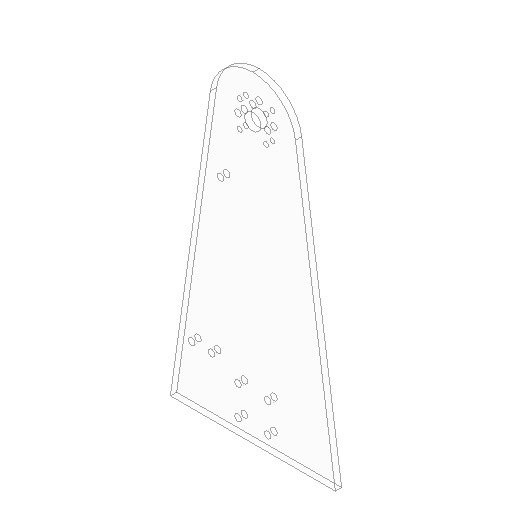
# Autodesk Inventor part: Columna
Saved by Autodesk Inventor 2025.3 (Build 293356000, 356)
## iProperties
Created: 2025-11-11
Part Number: Columna
Material: PMMA Plastic
Document SubType Name: Modeling
Designer: Gabriel Bojaca
Density: 1.188 g/cm^3
Appearance: Polycarbonate - Clear
Author: Gabriel Bojaca
Autodesk Inventor part; units mm, degrees
ref_plane "YZ Plane" through (0, 0, 0) normal (1, 0, 0) x (0, 1, 0)
ref_plane "XZ Plane" through (0, 0, 0) normal (0, 1, 0) x (-1, 0, 0)
ref_plane "XY Plane" through (0, 0, 0) normal (0, 0, 1) x (1, 0, 0)
sketch "Sketch3" plane through (0, 0, 0) normal (0, 0, 1) x (1, 0, 0)
  line L0 (0, 0) -> (100, 0)
  line L1 (100, 0) -> (100, 195) construction
  line L2 (100, 195) -> (0, 195) construction
  line L3 (0, 195) -> (0, 0) construction
  line L4 (50, 0) -> (50, 169) construction
  circle A0 centre (50, 169) radius 4.95
  line L5 (42, 161) -> (58, 161) construction
  line L6 (58, 161) -> (58, 177) construction
  line L7 (58, 177) -> (42, 177) construction
  line L8 (42, 177) -> (42, 161) construction
  line L9 (42, 161) -> (58, 177) construction
  line L10 (58, 161) -> (42, 177) construction
  circle A1 centre (42, 177) radius 1.5
  circle A2 centre (58, 177) radius 1.5
  circle A3 centre (42, 161) radius 1.5
  circle A4 centre (58, 161) radius 1.5
  line L11 (0, 0) -> (24.1871, 172.1)
  line L12 (0, 0) -> (268.3215, 0) construction
  line L13 (100, 0) -> (75.8129, 172.1)
  line L14 (0, 172.1) -> (100, 172.1) construction
  arc A5 (50, 195) -> (24.1871, 172.1) centre (50.5367, 168.3968) ccw
  arc A6 (75.8129, 172.1) -> (50, 195) centre (49.4633, 168.3968) ccw
  line L15 (50, 169) -> (59, 169) construction
  line L16 (50, 169) -> (41, 169) construction
  circle A7 centre (59, 169) radius 2
  circle A8 centre (41, 169) radius 2
  line L17 (41, 9) -> (59, 9) construction
  line L18 (59, 9) -> (59, 27) construction
  line L19 (59, 27) -> (41, 27) construction
  line L20 (41, 27) -> (41, 9) construction
  line L21 (41, 9) -> (59, 27) construction
  line L22 (59, 9) -> (41, 27) construction
  circle A9 centre (41, 27) radius 2
  circle A10 centre (41, 9) radius 2
  circle A11 centre (59, 27) radius 2
  circle A12 centre (59, 9) radius 2
  line L23 (50, 169) -> (50, 178) construction
  circle A13 centre (50, 178) radius 2
  point P0 (37.3431, 265.7102)
  point P1 (62.6569, 265.7102)
  point P2 (50, 18)
  dimension "d3" = 100
  dimension "d4" = 195
  dimension "d5" = 169
  dimension "d6" = 9.9
  dimension "d7" = 16
  dimension "d8" = 16
  dimension "d9" = 3
  dimension "d10" = 3
  dimension "d11" = 3
  dimension "d12" = 3
  dimension "d13" = 82
  dimension "d14" = 22.9
  dimension "d15" = 9
  dimension "d16" = 4
  dimension "d17" = 18
  dimension "d18" = 18
  dimension "d19" = 9
  dimension "d20" = 4
  dimension "d21" = 4
  dimension "d24" = 9
  dimension "d25" = 4
  constraints: 48 end point, 14 centre point, 9 coincident, 6 horizontal, 6 midpoint, 6 parallel, 6 point on line, 6 symmetric about line, 4 point on circle, 3 perpendicular, 1 tangent, 1 vertical, 4 other
  measures "d3" distance of L2.end L1.end
  measures "d4" distance of L1.end L0.end
  measures "d5" distance of L4.start L4.end
  measures "d6" diameter of A0
  measures "d7" distance of L7.end L6.end
  measures "d8" distance of L6.end L5.end
  measures "d9" diameter of A1
  measures "d10" diameter of A2
  measures "d11" diameter of A3
  measures "d12" diameter of A4
  measures "d13" angle of L12 L11
  measures "d14" distance between parallel lines of L14 L2
  measures "d15" distance of L15.start L15.end
  measures "d16" diameter of A7
  measures "d17" distance of L19.end L18.end
  measures "d18" distance of L18.end L17.end
  measures "d19" distance from line of L12 L17.start
  measures "d20" diameter of A9
  measures "d21" diameter of A10
  measures "d24" distance of L15.start L23.end
  measures "d25" diameter of A13
extrude "Extrusion2" add sketch "Sketch3" along normal blind 3.8
sketch "Sketch5" plane through (0, 0, 3.8) normal (0, 0, 1) x (1, 0, 0)
  circle A0 centre (-58.4959, 27.4361) radius 16.3248
  point P0 (0, 0)
  constraints: 1 centre point
sketch "Sketch6" plane through (0, 0, 3.8) normal (0, 0, 1) x (1, 0, 0)
  line L0 (177.5374, 0) -> (-44.6048, 0) construction
  line L1 (173.8282, 35) -> (-48.3141, 35) construction
  circle A0 centre (12.9189, 35) radius 2
  circle A1 centre (24.9189, 35) radius 2
  line L2 (24.1871, 172.1) -> (0, 0) projected
  point P0 (4.9189, 35)
  dimension "d33" = 35
  dimension "d34" = 4
  dimension "d35" = 4
  dimension "d36" = 12
  dimension "d37" = 8
  constraints: 4 end point, 4 point on line, 2 centre point, 1 horizontal, 1 parallel
  measures "d33" distance between parallel lines of L0 L1
  measures "d34" diameter of A0
  measures "d35" diameter of A1
  measures "d36" distance of A1.centre A0.centre
  measures "d37" distance of A0.centre point (4.919, 35)
extrude "Extrusion3" cut sketch "Sketch6" against normal blind 10
sketch "Sketch7" plane through (0, 0, 3.8) normal (0, 0, 1) x (1, 0, 0)
  line L0 (0, 0) -> (115.508, 0) construction
  line L1 (0, 130) -> (115.508, 130)
  line L2 (24.1871, 172.1) -> (0, 0) projected
  circle A0 centre (30.2703, 130) radius 2
  point P0 (18.2703, 130)
  dimension "d40" = 130
  dimension "d41" = 4
  dimension "d42" = 12
  constraints: 4 end point, 3 point on line, 1 centre point, 1 horizontal, 1 parallel
  measures "d40" distance between parallel lines of L0 L1
  measures "d41" diameter of A0
  measures "d42" distance of A0.centre point (18.27, 130)
extrude "Extrusion4" cut sketch "Sketch7" against normal blind 10
equation "\"d25\" = d16"
body "Solid2"
